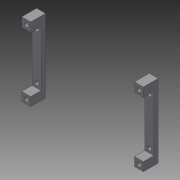
# Autodesk Inventor part: LCD_bracket
Saved by Autodesk Inventor 2015 (Build 190159000, 159)
## iProperties
Created: 2015-03-09
Part Number: LCD_bracket
Material: Generic
Document SubType Name: Modeling
Designer: ChristopherEvan
Density: 1 g/cm^3
Appearance: Default
Author: ChristopherEvan
Autodesk Inventor part; units mm, degrees
ref_plane "YZ Plane" through (0, 0, 0) normal (1, 0, 0) x (0, 1, 0)
ref_plane "XZ Plane" through (0, 0, 0) normal (0, 1, 0) x (-1, 0, 0)
sketch "Sketch1" plane through (0, 0, 0) normal (0, 0, 1) x (1, 0, 0)
  line L0 (75.25, 42.75) -> (75.25, -6.75)
  line L1 (75.25, -6.75) -> (81.25, -6.75)
  line L2 (81.25, -6.75) -> (81.25, 42.75)
  circle A0 centre (78.25, -3.75) radius 1.45
  circle A1 centre (78.25, 39.7484) radius 1.45
  circle A2 centre (78.25, 33.75) radius 1.45
  circle A3 centre (78.25, 2.25) radius 1.45
  line L3 (75.25, 42.75) -> (81.25, 42.75)
  line L4 (81.25, 42.75) -> (81.25, -6.75)
  line L5 (75.25, -6.75) -> (75.25, 42.75)
  line L6 (5.25, 18) -> (81.25, 18)
  line L7 (-0.75, 18) -> (81.25, 18)
  line L8 (40.25, 18) -> (40.25, 45.75)
  line L9 (40.25, 45.75) -> (40.25, 18)
  line L10 (40.25, -9.75) -> (40.25, 18)
  line L11 (75.25, 36.7484) -> (81.25, 36.7484)
  line L12 (75.25, -0.7484) -> (81.25, -0.7484)
  line L13 (5.25, 42.75) -> (5.25, -6.75)
  line L14 (5.25, -6.75) -> (-0.75, -6.75)
  line L15 (-0.75, -6.75) -> (-0.75, 42.75)
  circle A4 centre (2.25, -3.75) radius 1.45
  circle A5 centre (2.25, 39.7484) radius 1.45
  circle A6 centre (2.25, 33.75) radius 1.45
  circle A7 centre (2.25, 2.25) radius 1.45
  line L16 (5.25, 42.75) -> (-0.75, 42.75)
  line L17 (-0.75, 42.75) -> (-0.75, -6.75)
  line L18 (5.25, -6.75) -> (5.25, 42.75)
  line L19 (5.25, 36.7484) -> (-0.75, 36.7484)
  line L20 (5.25, -0.7484) -> (-0.75, -0.7484)
  line L21 (-13.8005, 43.9818) -> (170.3241, 43.9818)
  line L22 (-13.8005, -10.2335) -> (-13.8005, 43.9818)
  dimension "d9" = 18.7484
  dimension "d10" = 21.75
  dimension "d11" = 3
  constraints: 46 end point, 13 symmetric about line, 8 centre point, 3 equal length, 3 horizontal, 3 vertical, 2 midpoint, 1 perpendicular, 1 point on line, 7 other
  measures "d9" distance between parallel lines of L12 L6
  measures "d10" distance from line of L7 A0.centre
  measures "d11" distance from line of A0.centre L1
ref_plane "Work Plane1" through (0, 0, 3) normal (0, 0, 1) x (1, 0, 0)
extrude "Extrusion3" add sketch "Sketch1" along normal blind 3
sketch "Sketch4" plane through (0, 0, 0) normal (0, 0, -1) x (-1, 0, 0)
  line L0 (-81.25, 42.75) -> (-75.25, 42.75) projected
  circle A0 centre (-78.25, -3.75) radius 1.45 projected
  line L1 (-75.25, -6.75) -> (-81.25, -6.75) projected
  line L2 (-81.25, 42.75) -> (-75.25, 42.75)
  line L3 (-75.25, 42.75) -> (-75.25, 36.595)
  line L4 (-75.25, 36.595) -> (-81.25, 36.595)
  line L5 (-81.25, 36.595) -> (-81.25, 42.75)
  line L6 (-81.25, -6.75) -> (-75.25, -6.75)
  line L7 (-75.25, -6.75) -> (-75.25, -0.8339)
  line L8 (-75.25, -0.8339) -> (-81.25, -0.8339)
  line L9 (-81.25, -0.8339) -> (-81.25, -6.75)
  line L10 (-75.25, 18) -> (-5.25, 18)
  line L11 (-40.25, 18) -> (-40.25, 36.595)
  line L12 (-40.25, 36.595) -> (-40.25, 18)
  circle A1 centre (-78.25, 39.7484) radius 1.45 projected
  line L13 (0.75, 42.75) -> (-5.25, 42.75)
  line L14 (0.75, 42.75) -> (-5.25, 42.75)
  line L15 (-5.25, 42.75) -> (-5.25, 36.595)
  line L16 (-5.25, 36.595) -> (0.75, 36.595)
  line L17 (0.75, 36.595) -> (0.75, 42.75)
  circle A2 centre (-2.25, 39.7484) radius 1.45
  circle A3 centre (-2.25, -3.75) radius 1.45
  line L18 (-5.25, -6.75) -> (0.75, -6.75)
  line L19 (0.75, -6.75) -> (-5.25, -6.75)
  line L20 (-5.25, -6.75) -> (-5.25, -0.8339)
  line L21 (-5.25, -0.8339) -> (0.75, -0.8339)
  line L22 (0.75, -0.8339) -> (0.75, -6.75)
  constraints: 42 end point, 12 symmetric about line, 5 equal length, 2 centre point, 2 horizontal, 2 perpendicular, 1 midpoint, 1 vertical, 2 other
extrude "Extrusion4" add sketch "Sketch4" against normal blind 10
body "Solid2"
